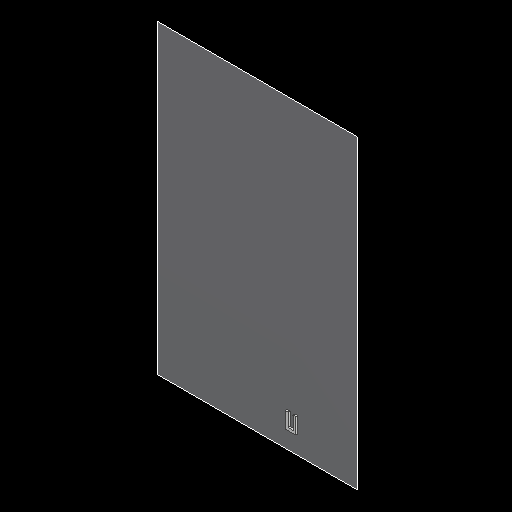
# Autodesk Inventor part: IRHolder_new2
Saved by Autodesk Inventor 2024.3 (Build 283343010, 343A)
## iProperties
Created: 2025-05-14
Part Number: IRHolder_new2
Material: Generic
Document SubType Name: Modeling
Designer: Oleg Kelner
Density: 1 g/cm^3
Appearance: Default
Author: Oleg Kelner
Autodesk Inventor part; units mm, degrees
ref_plane "YZ Plane" through (0, 0, 0) normal (1, 0, 0) x (0, 1, 0)
ref_plane "XZ Plane" through (0, 0, 0) normal (0, 1, 0) x (-1, 0, 0)
ref_plane "XY Plane" through (0, 0, 0) normal (0, 0, 1) x (1, 0, 0)
ref_plane "Work Plane2" through (0, 0, 0) normal (0, 0, 1) x (1, 0, 0)
sketch "Sketch2" plane through (0, 0, 0) normal (0, 0, 1) x (1, 0, 0)
  line L0 (-70.75, 49.5) -> (-69.25, 49.5) construction
  line L1 (-70.75, 39.5) -> (-70.75, 49.5) construction
  line L2 (-69.25, 39.5) -> (-70.75, 39.5) construction
  line L3 (-69.25, 49.5) -> (-69.25, 39.5) construction
  line L4 (-76.75, 49.5) -> (-75.25, 49.5) construction
  line L5 (-76.75, 39.5) -> (-76.75, 49.5) construction
  line L6 (-75.25, 39.5) -> (-76.75, 39.5) construction
  line L7 (-75.25, 39.5) -> (-75.25, 49.5) construction
  line L8 (-75.25, 44.5) -> (-70.75, 44.5) construction
  line L9 (-75.375, 39.5) -> (-75.375, 49.5)
  line L10 (-75.375, 49.5) -> (-70.625, 49.5) construction
  line L11 (-70.625, 49.5) -> (-70.625, 39.5)
  line L12 (-70.625, 39.5) -> (-75.375, 39.5)
  line L13 (-75.375, 39.5) -> (-70.625, 49.5) construction
  line L14 (-75.375, 49.5) -> (-70.625, 39.5) construction
  line L15 (-68, 37) -> (-78, 37)
  line L16 (-78, 37) -> (-78, 52)
  line L17 (-78, 52) -> (-75.375, 52)
  line L18 (-68, 52) -> (-68, 37)
  line L19 (-68, 37) -> (-78, 52) construction
  line L20 (-78, 37) -> (-68, 52) construction
  line L21 (-75.375, 49.5) -> (-75.375, 51)
  line L22 (-70.625, 49.5) -> (-70.625, 51)
  line L23 (-75.375, 52) -> (-70.625, 52) construction
  line L24 (-70.625, 52) -> (-68, 52)
  arc A0 (-75.375, 51) -> (-75.375, 52) centre (-75.375, 51.5) ccw
  arc A1 (-70.625, 52) -> (-70.625, 51) centre (-70.625, 51.5) ccw
  line L25 (-75.375, 51) -> (-75.375, 52) construction
  arc A2 (-75.375, 52) -> (-75.375, 51) centre (-75.375, 51.5) ccw construction
  arc A3 (-70.625, 51) -> (-70.625, 52) centre (-70.625, 51.5) ccw construction
  line L26 (-70.625, 51) -> (-70.625, 52) construction
  point P0 (0, 0)
  point P1 (-73, 44.5)
  dimension "d0" = 4.75
  dimension "d1" = 10
  dimension "d2" = 15
  dimension "d3" = 1
  dimension "d4" = 1
  constraints: 38 end point, 9 midpoint, 9 perpendicular, 8 point on circle, 6 parallel, 4 centre point, 4 point on line, 2 vertical, 1 horizontal
  measures "d0" distance of L9.end L10.end
  measures "d1" distance of L15.start L15.end
  measures "d2" distance of L15.end L16.end
  measures "d3" diameter of A0
  measures "d4" diameter of A1
extrude "Extrusion1" add sketch "Sketch2" along normal blind 1.9
body "Solid1"
